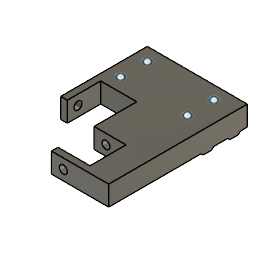
Fixed Roller Bracket B (Autodesk Fusion 360 design; units mm, degrees)
part number: 2026-05-27-15-50-34-677
Autodesk Fusion 360 part; units mm, degrees
note: some values were not read from the file. Set by a fixed rule: which sketch regions a step uses.
sketch "Sketch1" plane through (0, 0, 0) normal (0, 0, 1) x (1, 0, 0)
  line L0 (-25, -15) -> (-25, 50)
  line L1 (-25, 50) -> (50, 50)
  line L2 (50, 50) -> (50, -54)
  line L3 (-20, -15) -> (-20, 10)
  line L4 (-20, 10) -> (7, 10)
  line L5 (7, -22) -> (7, 10)
  line L6 (-19, -7) -> (6, -7)
  line L7 (-25, -15) -> (-20, -15)
  line L8 (7, -22) -> (31, -22)
  line L9 (16, -23) -> (16, -48)
  line L10 (-19, -20) -> (6, -20) construction
  line L11 (-19, 6) -> (6, 6) construction
  line L12 (29, -23) -> (29, -48) construction
  line L13 (31, -22) -> (31, -49)
  line L14 (7, -49) -> (31, -49)
  line L15 (7, -54) -> (50, -54)
  line L16 (7, -49) -> (7, -54)
  circle A0 centre (-15, 20) radius 2.7
  circle A1 centre (35, 20) radius 2.7
  circle A2 centre (-15, 40) radius 2.7
  circle A3 centre (35, 40) radius 2.7
  line L17 (3, -23) -> (3, -48) construction
  line L18 (3, -23) -> (29, -23) construction
  line L19 (3, -48) -> (29, -48) construction
  line L20 (-19, 6) -> (-19, -20) construction
  line L21 (6, 6) -> (6, -20) construction
  dimension "d10" = 5.4
  dimension "d13" = 50
  dimension "d14" = 20
  dimension "d35" = 25
  dimension "d36" = 1
  dimension "d37" = 25
  dimension "d38" = 1
  dimension "d39" = 65
  constraint parallel L0 L2
  constraint perpendicular L3 L7
  constraint perpendicular L5 L8
  constraint perpendicular L8 L9
  constraint perpendicular L15 L16
  constraint perpendicular L12 L18
  constraint perpendicular L12 L19
  constraint perpendicular L10 L20
  constraint perpendicular L10 L21
  constraint coincident L6.start L20
  constraint coincident L6.end L21
  constraint coincident L9.start L18
  constraint coincident L9.end L19
  measures "d10" diameter of A0
  measures "d35" distance of L9.start L9.end
  measures "d36" distance of L8 L9.start
  measures "d37" distance of L6.start L6.end
  measures "d38" distance of L5 L6.end
  measures "d39" distance of L1 L7
extrude "Extrude1" add sketch "Sketch1" along normal blind 15
sketch "Sketch2" plane through (-25, 0, 0) normal (-1, 0, 0) x (0, -1, 0)
  circle A0 centre (7, 7.5) radius 3
  dimension "d17" = 6
  measures "d17" diameter of A0
sketch "Sketch4" plane through (0, -54, 0) normal (0, -1, 0) x (1, 0, 0)
  circle A0 centre (16, 7.5) radius 3
  dimension "d18" = 6
  measures "d18" diameter of A0
extrude "Extrude2" cut sketch "Sketch2" against normal blind 40
extrude "Extrude3" cut sketch "Sketch4" against normal blind 40
sketch "Sketch5" plane through (-25, 0, 0) normal (-1, 0, 0) x (0, -1, 0)
  line L0 (-24.8003, 0) -> (-15.2003, 0)
  line L1 (-44.8003, 0) -> (-35.2003, 0)
  line L2 (-23.2003, -1.6) -> (-16.8003, -1.6)
  line L3 (-43.2003, -1.6) -> (-36.8003, -1.6)
  line L4 (-43.2003, -1.6) -> (-44.8003, 0)
  line L5 (-36.8003, -1.6) -> (-35.2003, 0)
  line L6 (-23.2003, -1.6) -> (-24.8003, 0)
  line L7 (-16.8003, -1.6) -> (-15.2003, 0)
extrude "Extrude4" add sketch "Sketch5" against normal blind 75
sketch "Sketch6" plane through (0, 0, 15) normal (0, 0, 1) x (-1, 0, 0)
  circle A0 centre (15, -40) radius 2.7
  circle A1 centre (15, -20) radius 2.7
  circle A2 centre (-35, -20) radius 2.7
  circle A3 centre (-35, -40) radius 2.7
extrude "Extrude5" cut sketch "Sketch6" against normal blind 20
named bodies: "Fixed Roller Bracket B"
